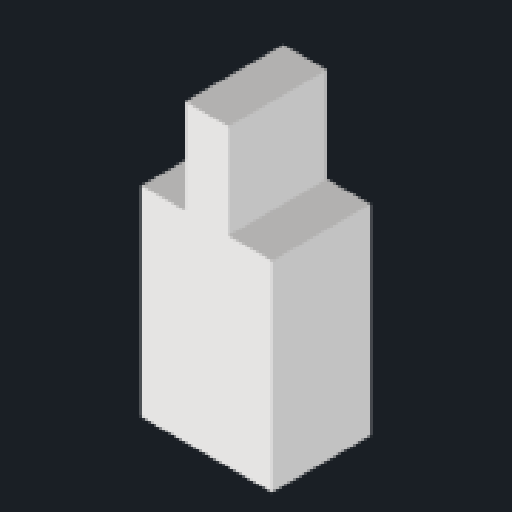
# Autodesk Inventor part: ForearmActuatorConnectorBoundingBox
Saved by Autodesk Inventor 2023 (Build 270158000, 158)
## iProperties
Created: 2023-03-28
Part Number: ForearmActuatorConnectorBoundingBox
Material: Generic
Document SubType Name: Modeling
Designer: LattePanda
Density: 1 g/cm^3
Appearance: Default
Author: LattePanda
Autodesk Inventor part; units mm, degrees
ref_plane "YZ Plane" through (0, 0, 0) normal (1, 0, 0) x (0, 1, 0)
ref_plane "XZ Plane" through (0, 0, 0) normal (0, 1, 0) x (-1, 0, 0)
sketch "Sketch1" plane through (0, 0, 0) normal (0, 0, 1) x (1, 0, 0)
  line L0 (-2.81, 5) -> (2.81, 5)
  line L1 (2.81, 5) -> (2.81, -33.1)
  line L2 (2.81, -33.1) -> (-2.81, -33.1)
  line L3 (-2.81, -33.1) -> (-2.81, 5)
  line L4 (-2.81, -33.1) -> (-8.43, -33.1)
  line L5 (-8.43, -33.1) -> (-8.43, -7.2065)
  line L6 (-8.43, -7.2065) -> (-2.81, -7.2065)
  line L7 (-2.81, -7.2065) -> (-2.81, -33.1)
  line L8 (-13.3844, -4.6707) -> (3.9886, -4.5258) construction
  line L9 (4.1365, -22.2635) -> (-13.2364, -22.4084) construction
  line L10 (-18.4107, -1.5425) -> (-18.3842, -4.7124) construction
  line L11 (42.6603, -9.7914) -> (42.6338, -6.6215) projected
  line L12 (0, -40.72) -> (0, 12.62) construction
  line L13 (2.81, -33.1) -> (8.43, -33.1)
  line L14 (8.43, -33.1) -> (8.43, -7.2065)
  line L15 (8.43, -7.2065) -> (2.81, -7.2065)
  line L16 (2.81, -7.2065) -> (2.81, -33.1)
  point P0 (0, 0)
  point P1 (42.647, -8.2065)
  dimension "d0" = 1
  dimension "d1" = 1
  dimension "d2" = 1
  dimension "d3" = 38.1
  dimension "d4" = 1
  constraints: 24 end point, 4 parallel, 3 symmetric about line, 2 horizontal, 2 perpendicular, 1 collinear, 1 midpoint
  measures "d3" distance of L2.end L0.start
  measures "d4" distance from line of point (42.647, -8.206) L6
ref_plane "Work Plane1" through (6.228, -54, -6.35) normal (0, 0, -1) x (0, 1, 0)
extrude "Extrusion1" add sketch "Sketch1" along normal mid plane 12.7
body "Solid1"
